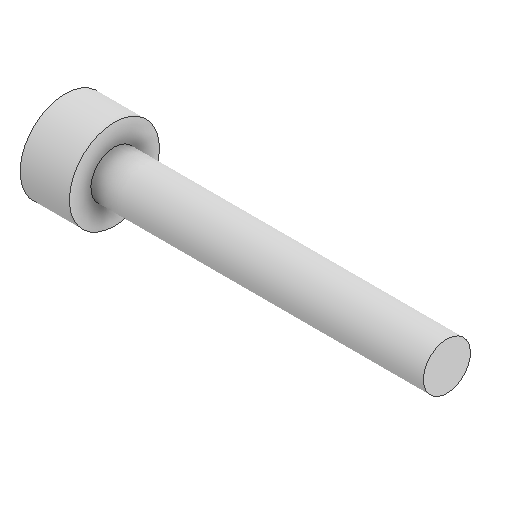
# Autodesk Inventor part: Screw PROP
Saved by Autodesk Inventor 2025 (Build 290162010, 162A)
## iProperties
Created: 2024-12-04
Part Number: Screw PROP
Material: Generic
Document SubType Name: Modeling
Designer: ALEXANDERNICHOLS
Density: 1 g/cm^3
Appearance: Default
Author: ALEXANDERNICHOLS
Autodesk Inventor part; units mm, degrees
ref_plane "YZ Plane" through (0, 0, 0) normal (1, 0, 0) x (0, 1, 0)
ref_plane "XZ Plane" through (0, 0, 0) normal (0, 1, 0) x (-1, 0, 0)
ref_plane "XY Plane" through (0, 0, 0) normal (0, 0, 1) x (1, 0, 0)
sketch "Sketch1" plane through (0, 0, 0) normal (0, 0, 1) x (1, 0, 0)
  line L0 (0, 0) -> (0, 1.397)
  line L1 (0, 1.397) -> (-19.7104, 1.397)
  line L2 (-19.7104, 1.397) -> (-19.7104, 2.667)
  line L3 (-19.7104, 2.667) -> (-22.6314, 2.667)
  line L4 (-22.6314, 2.667) -> (-22.6314, 0)
  line L5 (-22.6314, 0) -> (0, 0)
  point P0 (-19.7104, 2.032)
  dimension "d0" = 5.334
  dimension "d1" = 2.794
  dimension "d2" = 2.921
  dimension "d3" = 19.7104
  constraints: 12 end point, 5 perpendicular, 1 midpoint, 1 vertical
  measures "d0" diameter of L3 L5
  measures "d1" diameter of L1 L5
  measures "d2" distance from line of L4 point (-19.71, 2.032)
  measures "d3" distance of L0.end L1.end
revolve "Revolution1" add sketch "Sketch1" angle 360 about axis through (-22.6314, 0, 0) along (1, 0, 0)
body "Solid1"
